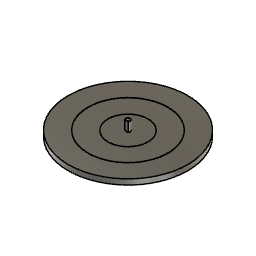
Encoder-Optico-Circ v7 (Autodesk Fusion 360 design; units mm, degrees)
Autodesk Fusion 360 part; units mm, degrees
sketch "Esboço1" plane through (0, 0, 0) normal (0, 0, 1) x (1, 0, 0)
  circle A0 centre (0, 0) radius 50
  circle A1 centre (0, 0) radius 33.33
  circle A2 centre (0, 0) radius 16.7
  line L0 (-1.4867, -1.3378) -> (1.4867, -1.3378)
  arc A3 (1.4867, -1.3378) -> (-1.4867, -1.3378) centre (0, 0) ccw
  arc A4 (1.3948, -1.1378) -> (-1.3948, -1.1378) centre (0, 0) ccw
  line L1 (-1.3948, -1.1378) -> (1.3948, -1.1378)
  dimension "d1" = 100
  dimension "d5" = -16.67
  dimension "d6" = -33.3
  dimension "d7" = 4
  dimension "d18" = -0.2
  constraint coincident A0.centre A1.centre
  constraint concentric A0 A3
  constraint horizontal L0
  measures "d1" diameter of A0
  measures "d7" diameter of A3
extrude "Extrusão1" add sketch "Esboço1" along normal blind 0.5 contours A0 makes body 1
extrude "Extrusão2" add sketch "Esboço1" along normal blind 0.3 contours A1 bodies 1
extrude "Extrusão3" add sketch "Esboço1" along normal blind 0.2 contours A2 bodies 1
extrude "Extrusão7" cut sketch "Esboço1" along normal blind 0.5 contours L0 A3 bodies 1
extrude "Extrusão6" add sketch "Esboço1" along normal blind 15 separate body contours A4 L1 makes body 2
move_body "Mover2" bodies 2 to x (1, 0, 0) y (0, 1, 0) z (0, 0, 1) at (60, 0, 0)
shell "Casca1" thickness 0.2 removed faces 1 at (60.3061, 0.1512, 15) on bodies 2
extrude "Extrusão8" add 1 faces at (44.1331, -4.1399, 0.5) along direction (0, 0, 1) blind 4 on bodies 1 bodies 1
extrude "Extrusão9" add 1 faces at (27.6004, -2.4855, 0.3) along direction (0, 0, 1) blind 4 on bodies 1 bodies 1
extrude "Extrusão10" add 1 faces at (-0.416, -6.443, 0.2) along direction (0, 0, 1) blind 4 on bodies 1 bodies 1
extrude "Extrusão11" add sketch "Esboço1" along normal blind 12 contours L0 A3 bodies 1
hidden bodies 2
